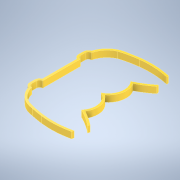
# Autodesk Inventor part: ovladac
Saved by Autodesk Inventor 2022 (Build 260153000, 153)
## iProperties
Created: 2022-12-02
Part Number: ovladac
Material: Generic
Document SubType Name: Modeling
Designer: matys
Density: 1 g/cm^3
Appearance: Glossy - Gold
Author: matys
Autodesk Inventor part; units mm, degrees
ref_plane "YZ Plane" through (0, 0, 0) normal (1, 0, 0) x (0, 1, 0)
ref_plane "XZ Plane" through (0, 0, 0) normal (0, 1, 0) x (-1, 0, 0)
ref_plane "XY Plane" through (0, 0, 0) normal (0, 0, 1) x (1, 0, 0)
sketch "Sketch1" plane through (0, 0, 0) normal (0, 1, 0) x (-1, 0, 0)
  circle A0 centre (0, 0) radius 17.5
  line L0 (0, -17.5) -> (0, -77.5)
  line L1 (0, -77.5) -> (0, -95)
  circle A1 centre (0, -95) radius 17.5
  line L2 (0, 0) -> (0, -25)
  line L3 (0, -25) -> (-22.5, -25)
  circle A2 centre (-22.5, -25) radius 12.5
  line L4 (-86.0476, -189.7218) -> (-86.0476, -216.7218)
  line L5 (-86.0476, -216.7218) -> (-52.0476, -216.7218)
  line L6 (-52.0476, -216.7218) -> (-52.0476, -189.7218)
  line L7 (-52.0476, -189.7218) -> (-86.0476, -189.7218)
  line L8 (-86.0476, -189.7218) -> (-52.0476, -216.7218)
  line L9 (-52.0476, -189.7218) -> (-86.0476, -216.7218)
  line L10 (0, -25) -> (0, -17.5)
  line L11 (0, -25) -> (0, -32.5)
  circle A3 centre (-22.5, -70) radius 12.5
  line L12 (-39.5, -56.5) -> (-39.5, -83.5)
  line L13 (-39.5, -83.5) -> (-5.5, -83.5)
  line L14 (-5.5, -83.5) -> (-5.5, -56.5)
  line L15 (-5.5, -56.5) -> (-39.5, -56.5)
  line L16 (-39.5, -56.5) -> (-5.5, -83.5)
  line L17 (-5.5, -56.5) -> (-39.5, -83.5)
  line L18 (-5.5, -56.5) -> (-22.5, -70)
  line L19 (-109.6323, -189.7218) -> (-115.6323, -189.7218)
  line L20 (-115.6323, -189.7218) -> (-115.6323, -195.7218)
  line L21 (-115.6323, -195.7218) -> (-109.6323, -195.7218)
  line L22 (-109.6323, -195.7218) -> (-109.6323, -189.7218)
  line L23 (-115.6323, -189.7218) -> (-109.6323, -195.7218)
  line L24 (-109.6323, -189.7218) -> (-115.6323, -195.7218)
  line L25 (0, -112.5) -> (0, -106)
  line L26 (-3, -109) -> (-3, -103)
  line L27 (-3, -103) -> (3, -103)
  line L28 (3, -103) -> (3, -109)
  line L29 (3, -109) -> (-3, -109)
  line L30 (14, -98) -> (8, -98)
  line L31 (14, -92) -> (14, -98)
  line L32 (8, -98) -> (8, -92)
  line L33 (8, -92) -> (14, -92)
  line L34 (3, -81) -> (3, -87)
  line L35 (-3, -81) -> (3, -81)
  line L36 (3, -87) -> (-3, -87)
  line L37 (-3, -87) -> (-3, -81)
  line L38 (-14, -92) -> (-8, -92)
  line L39 (-14, -98) -> (-14, -92)
  line L40 (-8, -92) -> (-8, -98)
  line L41 (-8, -98) -> (-14, -98)
  line L42 (-135.6088, -189.7218) -> (-135.6088, -214.7218)
  line L43 (-135.6088, -214.7218) -> (-162.6088, -214.7218)
  line L44 (-162.6088, -214.7218) -> (-162.6088, -189.7218)
  line L45 (-162.6088, -189.7218) -> (-135.6088, -189.7218)
  line L46 (-162.6088, -189.7218) -> (-135.6088, -214.7218)
  line L47 (-135.6088, -189.7218) -> (-162.6088, -214.7218)
  line L48 (17.5, 0) -> (17.5, -95)
  line L49 (-162.6088, -202.2218) -> (-135.6088, -202.2218)
  line L50 (25.5, -35) -> (25.5, -60)
  line L51 (25.5, -60) -> (-1.5, -60)
  line L52 (-1.5, -60) -> (-1.5, -35)
  line L53 (-1.5, -35) -> (25.5, -35)
  line L54 (25.5, -35) -> (20.5, -35)
  line L55 (20.5, -35) -> (20.5, -60)
  line L56 (-1.5, -35) -> (6.5, -35)
  line L57 (6.5, -35) -> (6.5, -60)
  line L58 (-1.5, -47.5) -> (6.5, -47.5)
  line L59 (-1.5, -35) -> (35.8, -35)
  line L60 (25.5, -60) -> (29.5, -60)
  line L61 (29.5, -60) -> (29.5, -47.5)
  line L62 (29.5, -47.5) -> (25.5, -47.5)
  line L63 (29.5, -60) -> (-7.8, -60)
  line L64 (-7.8, -60) -> (-7.8, -35)
  line L65 (-7.8, -35) -> (-1.5, -35)
  dimension "d0" = 35
  dimension "d1" = 60
  dimension "d2" = 17.5
  dimension "d3" = 25
  dimension "d4" = 22.5
  dimension "d6" = 25
  dimension "d7" = 27
  dimension "d8" = 34
  dimension "d9" = 27
  dimension "d10" = 7.5
  dimension "d11" = 25
  dimension "d12" = 27
  dimension "d13" = 34
  dimension "d14" = 27
  dimension "d15" = 6
  dimension "d16" = 6
  dimension "d17" = 6
  dimension "d18" = 6.5
  dimension "d22" = 6
  dimension "d25" = 360
  dimension "d27" = 25
  dimension "d28" = 27
  dimension "d32" = 25
  dimension "d33" = 27
  dimension "d34" = 5
  dimension "d35" = 8
  dimension "d36" = 8
  dimension "d72" = 37.3
  dimension "d73" = 4
  dimension "d74" = 37.3
  constraints: 132 end point, 20 perpendicular, 8 point on line, 8 vertical, 6 midpoint, 5 point on circle, 4 centre point, 3 coincident, 3 horizontal, 1 collinear, 1 tangent, 33 other
  measures "d0" diameter of A0
  measures "d1" distance of L0.start L0.end
  measures "d2" distance of L0.end L1.end
  measures "d3" distance of L2.start L2.end
  measures "d4" distance of L2.end L3.end
  measures "d6" diameter of A2
  measures "d7" distance of L4.start L4.end
  measures "d8" distance of L4.end L5.end
  measures "d9" distance of L5.end L6.end
  measures "d10" distance of L2.end L11.end
  measures "d11" diameter of A3
  measures "d12" distance of L15.end L12.end
  measures "d13" distance of L12.end L14.start
  measures "d14" distance of L14.start L15.start
  measures "d15" distance of L19.start L19.end
  measures "d16" distance of L19.end L20.end
  measures "d17" distance of L20.end L21.end
  measures "d18" distance of L25.start L25.end
  measures "d22" distance of L26.start L26.end
  measures "d27" distance of L42.start L42.end
  measures "d28" distance of L42.end L43.end
  measures "d32" distance of L50.start L50.end
  measures "d33" distance of L50.end L51.end
  measures "d34" distance of L50.start L54.end
  measures "d35" distance of L52.end L56.end
  measures "d36" distance between parallel lines of L50 L48
  measures "d72" distance of L52.end L59.end
  measures "d73" distance of L50.end L60.end
  measures "d74" distance of L60.end L63.end
sketch "Sketch2" plane through (0, 0, 0) normal (0, 1, 0) x (-1, 0, 0)
  circle A0 centre (0, 0) radius 17.5
  line L0 (0, 17.5) -> (0, 25.5)
  line L1 (17.5, 0) -> (29.5, 0)
  line L2 (0, 0) -> (0, 17.5)
  line L3 (0, 17.5) -> (17.5, 0)
  line L4 (0, 0) -> (8.75, 8.75)
  line L5 (8.75, 8.75) -> (12.3744, 12.3744)
  line L6 (12.3744, 12.3744) -> (18.0312, 18.0312)
  arc A1 (29.5, 0) -> (10.5727, 22.6518) centre (-3.4308, -8.2827) ccw
  line L7 (0, -20.5) -> (0, -80.5)
  line L8 (0, -80.5) -> (0, -98)
  line L9 (29.5, 0) -> (29.5, -17.5) construction
  line L10 (34.5, -12.5) -> (34.5, -5)
  arc A2 (34.5, -5) -> (29.5, 0) centre (29.5, -5) ccw
  arc A3 (29.5, -17.5) -> (34.5, -12.5) centre (29.5, -12.5) ccw
  line L11 (29.5, -17.5) -> (29.5, -47.5)
  line L12 (0, -20.5) -> (0, -25.5)
  line L13 (0, -17.5) -> (0, -21.5)
  line L14 (0, -17.5) -> (0, -25)
  line L15 (0, -25) -> (-22.5, -25)
  circle A4 centre (-22.5, -25) radius 12.5
  line L16 (-9, -8) -> (-36, -8)
  line L17 (-36, -8) -> (-36, -42)
  line L18 (-36, -42) -> (-9, -42)
  line L19 (-9, -42) -> (-9, -8)
  line L20 (-36, -42) -> (-9, -8)
  line L21 (-36, -8) -> (-9, -42)
  line L22 (-22.5, -25) -> (-36, -42)
  line L23 (0, -17.5) -> (0, -11)
  line L24 (0, -11) -> (3, -11)
  line L25 (3, -11) -> (3, -8)
  line L26 (3, -8) -> (-3, -8)
  line L27 (-3, -8) -> (-3, -14)
  line L28 (-3, -14) -> (3, -14)
  line L29 (3, -14) -> (3, -11)
  line L30 (14, 3) -> (11, 3)
  line L31 (8, 3) -> (8, -3)
  line L32 (11, 3) -> (8, 3)
  line L33 (8, -3) -> (14, -3)
  line L34 (14, -3) -> (14, 3)
  line L35 (-3, 14) -> (-3, 11)
  line L36 (-3, 8) -> (3, 8)
  line L37 (-3, 11) -> (-3, 8)
  line L38 (3, 8) -> (3, 14)
  line L39 (3, 14) -> (-3, 14)
  line L40 (-14, -3) -> (-11, -3)
  line L41 (-8, -3) -> (-8, 3)
  line L42 (-11, -3) -> (-8, -3)
  line L43 (-8, 3) -> (-14, 3)
  line L44 (-14, 3) -> (-14, -3)
  line L45 (0, -47.5) -> (-33.3972, -47.5)
  arc A5 (-41.1706, -8.3745) -> (-33.3972, -47.5) centre (-22.5, -25) ccw
  arc A6 (10.5727, -117.6518) -> (29.5, -95) centre (-3.4308, -86.7173) ccw
  line L46 (34.5, -82.5) -> (34.5, -90)
  arc A7 (29.5, -95) -> (34.5, -90) centre (29.5, -90) ccw
  arc A8 (34.5, -82.5) -> (29.5, -77.5) centre (29.5, -82.5) ccw
  line L47 (29.5, -77.5) -> (29.5, -47.5)
  ellipse E0 centre (-5.5218, -98.3783) end of major axis (-65.9225, -112.4065) minor radius 22.7978 (-28.0257, -81.2123) -> (10.5727, -117.6518) ccw
  arc A9 (-33.3972, -47.5) -> (-41.1706, -86.6255) centre (-22.5, -70) ccw
  line L48 (0, -95) -> (0, -112.5)
  line L49 (-9, -87) -> (-36, -87)
  line L50 (-36, -87) -> (-36, -53)
  line L51 (-36, -53) -> (-9, -53)
  line L52 (-9, -53) -> (-9, -87)
  line L53 (0, -77.5) -> (0, -84)
  line L54 (0, -84) -> (3, -84)
  line L55 (3, -84) -> (3, -87)
  line L56 (3, -87) -> (-3, -87)
  line L57 (-3, -87) -> (-3, -81)
  line L58 (-3, -81) -> (3, -81)
  line L59 (3, -81) -> (3, -84)
  line L60 (14, -98) -> (11, -98)
  line L61 (8, -98) -> (8, -92)
  line L62 (11, -98) -> (8, -98)
  line L63 (8, -92) -> (14, -92)
  line L64 (14, -92) -> (14, -98)
  line L65 (-3, -109) -> (-3, -106)
  line L66 (-3, -103) -> (3, -103)
  line L67 (-3, -106) -> (-3, -103)
  line L68 (3, -103) -> (3, -109)
  line L69 (3, -109) -> (-3, -109)
  line L70 (-14, -92) -> (-11, -92)
  line L71 (-8, -92) -> (-8, -98)
  line L72 (-11, -92) -> (-8, -92)
  line L73 (-8, -98) -> (-14, -98)
  line L74 (-14, -98) -> (-14, -92)
  line L75 (0, -47.5) -> (-1.5, -47.5)
  line L76 (-1.5, -47.5) -> (-1.5, -60)
  line L77 (-1.5, -60) -> (25.5, -60)
  line L78 (25.5, -60) -> (25.5, -35)
  line L79 (25.5, -35) -> (-1.5, -35)
  line L80 (-1.5, -35) -> (-1.5, -47.5)
  line L81 (0, -17.5) -> (0, -25)
  line L82 (0, -47.5) -> (0, -35)
  line L83 (25.5, -44.7664) -> (24.099, -44.7664)
  line L84 (-5.5218, 3.3783) -> (-65.9225, 17.4065)
  line L85 (-5.5218, 3.3783) -> (-5.5218, 9.5)
  line L86 (-65.9225, 17.4065) -> (128.8922, -27.8397)
  line L87 (0, 0) -> (0, -15)
  line L88 (0, -15) -> (15, -15)
  line L89 (15, -15) -> (15, 15)
  line L90 (15, 15) -> (-15, 15)
  line L91 (-15, 15) -> (-15, -15)
  line L92 (0, -15) -> (-15, -15)
  line L93 (-65.9225, 17.4065) -> (-19.167, 6.5474)
  line L94 (-19.167, 6.5474) -> (-21.2031, -2.2192)
  line L95 (-21.2031, -2.2192) -> (-67.9586, 8.6399)
  line L96 (-67.9586, 8.6399) -> (-65.9225, 17.4065)
  line L97 (-65.9225, 17.4065) -> (-63.8865, 26.1732)
  line L98 (-63.8865, 26.1732) -> (-17.1309, 15.3141)
  line L99 (-17.1309, 15.3141) -> (-19.167, 6.5474)
  line L100 (-21.2031, -2.2192) -> (-28.0257, -13.7877)
  line L101 (-28.0257, -13.7877) -> (-21.0551, 16.2255)
  arc A10 (-67.9586, 8.6399) -> (-28.0257, -13.7877) centre (15.2695, 110.0655) ccw
  line L102 (-28.0257, -13.7877) -> (-21.0551, 16.2255)
  arc A11 (-18.1566, 28.7053) -> (-63.8865, 26.1732) centre (-33.8791, -101.5517) ccw
  line L103 (-63.8865, 26.1732) -> (-65.0129, 25.9033)
  line L104 (-67.9586, 8.6399) -> (-68.8508, 9.3786)
  ellipse E1 centre (-65.9225, 17.4065) end of major axis (-63.8865, 26.1732) minor radius 3.0998 (-67.9586, 8.6399) -> (-63.8865, 26.1732) ccw
  ellipse E2 centre (-65.9225, 17.4065) end of major axis (-63.8865, 26.1732) minor radius 3.0998 (-65.0129, 25.9033) -> (-68.8508, 9.3786) ccw
  line L105 (-67.9586, 8.6399) -> (-67.2799, 11.5621)
  line L106 (-67.2799, 11.5621) -> (-64.3577, 10.8834)
  line L107 (-64.3577, 10.8834) -> (-65.0364, 7.9612)
  line L108 (-63.8865, 26.1732) -> (-64.5652, 23.251)
  line L109 (-64.5652, 23.251) -> (-63.8865, 26.1732)
  line L110 (-63.8865, 26.1732) -> (-60.9642, 25.4945)
  line L111 (-60.9642, 25.4945) -> (-61.6429, 22.5723)
  line L112 (-61.6429, 22.5723) -> (-64.5652, 23.251)
  line L113 (0, -80) -> (15, -80)
  line L114 (15, -80) -> (15, -110)
  line L115 (15, -110) -> (-15, -110)
  line L116 (-15, -110) -> (-15, -80)
  line L117 (0, -80) -> (-15, -80)
  arc A12 (-28.0257, -81.2123) -> (-67.9586, -103.6399) centre (15.2695, -205.0655) ccw
  arc A13 (-63.8865, -121.1732) -> (-18.1566, -123.7053) centre (-33.8791, 6.5517) ccw
  line L118 (-63.8865, -121.1732) -> (-65.0129, -120.9033)
  line L119 (-67.9586, -103.6399) -> (-68.8508, -104.3786)
  ellipse E3 centre (-65.9225, -112.4065) end of major axis (-63.8865, -121.1732) minor radius 3.0998 (-68.8508, -104.3786) -> (-65.0129, -120.9033) ccw
  line L120 (0, -47.5) -> (6.5, -47.5)
  line L121 (6.5, -47.5) -> (6.5, -60)
  line L122 (6.5, -60) -> (6.5, -80)
  line L123 (6.5, -70) -> (6.5, -60)
  line L124 (6.5, -60) -> (20.5, -60)
  line L125 (20.5, -60) -> (20.5, -70)
  line L126 (20.5, -70) -> (6.5, -70)
  line L127 (6.5, -70) -> (6.5, -67)
  line L128 (6.5, -67) -> (8, -67)
  line L129 (8, -67) -> (8, -70)
  line L130 (8, -67) -> (20.5, -67)
  line L131 (20.5, -67) -> (19, -67)
  line L132 (19, -67) -> (19, -70)
  line L133 (6.5, -60) -> (6.5, -70)
  line L134 (6.5, -70) -> (6.5, -73)
  line L135 (6.5, -73) -> (19, -73)
  line L136 (19, -73) -> (19, -70)
  line L137 (8, -73) -> (8, -70)
  line L138 (19, -70) -> (8, -70)
  line L139 (8, -28) -> (8, -25)
  line L140 (8, -28) -> (20.5, -28)
  line L141 (19, -28) -> (19, -25)
  line L142 (6.5, -22) -> (19, -22)
  line L143 (19, -22) -> (19, -25)
  line L144 (8, -22) -> (8, -25)
  line L145 (25.5, -60) -> (25.5, -73)
  line L146 (25.5, -73) -> (19, -73)
  ellipse E4 centre (-5.5218, 3.3783) end of major axis (-65.9225, 17.4065) minor radius 22.7978 (10.5727, 22.6518) -> (-18.1566, 28.7053) ccw
  ellipse E5 centre (-5.5218, 3.3783) end of major axis (-65.9225, 17.4065) minor radius 22.7978 (-58.9806, 25.0338) -> (-64.5851, 9.9042) ccw
  ellipse E6 centre (-5.5218, 3.3783) end of major axis (-65.9225, 17.4065) minor radius 22.7978 (-63.0527, 7.5005) -> (-28.0257, -13.7877) ccw
  arc A14 (-17.8019, 31.6843) -> (-63.1315, 29.4239) centre (-33.8791, -101.5517) ccw
  line L147 (-18.1328, 15.5468) -> (-25.1035, -14.4663)
  arc A15 (31.8748, 2.6394) -> (0.4994, 28.4642) centre (-3.4308, -8.2827) ccw
  line L148 (25.5, -47.5) -> (29.5, -47.5)
  line L149 (32.5, -47.5) -> (32.5, -19.9162)
  arc A16 (32.5, -19.9162) -> (37.5, -12.5) centre (29.5, -12.5) ccw
  line L150 (37.5, -12.5) -> (37.5, -5)
  arc A17 (37.5, -5) -> (31.8748, 2.6394) centre (29.5, -5) ccw
  line L151 (-65.9225, 17.4065) -> (-63.1315, 29.4239)
  arc A18 (-68.7136, 5.3892) -> (-45.7824, -9.4458) centre (15.2695, 110.0655) ccw
  arc A19 (-43.9451, -6.997) -> (-43.9554, -7.0092) centre (-22.5, -25) ccw
  arc A20 (-45.7824, -9.4458) -> (-39.1658, -47.5) centre (-22.5, -25) ccw
  line L152 (-65.9225, 17.4065) -> (-68.7136, 5.3892)
  arc A21 (-45.7824, -85.5542) -> (-68.7136, -100.3892) centre (15.2695, -205.0655) ccw
  arc A22 (-39.1658, -47.5) -> (-45.7824, -85.5542) centre (-22.5, -70) ccw
  line L153 (-65.9225, -112.4065) -> (-68.7136, -100.3892)
  arc A23 (-63.1315, -124.4239) -> (-17.8019, -126.6843) centre (-33.8791, 6.5517) ccw
  arc A24 (0.4994, -123.4642) -> (31.8748, -97.6394) centre (-3.4308, -86.7173) ccw
  line L154 (32.5, -47.5) -> (32.5, -75.0838)
  arc A25 (37.5, -82.5) -> (32.5, -75.0838) centre (29.5, -82.5) ccw
  line L155 (37.5, -82.5) -> (37.5, -90)
  arc A26 (31.8748, -97.6394) -> (37.5, -90) centre (29.5, -90) ccw
  line L156 (-65.9225, -112.4065) -> (-63.1315, -124.4239)
  arc A27 (-17.8019, -126.6843) -> (0.4994, -123.4642) centre (-51.4005, 117.889) ccw
  spline S0 degree 5 poles (-17.8067, 31.6848) (-14.1127, 31.2511) (-10.4318, 30.7055) (-6.7676, 30.0569) (-3.1227, 29.3096) (0.4994, 28.4642) knots 0 0 0 0 0 0 1 1 1 1 1 1
  point P0 (29.5, -8.75)
  point P1 (0, -35)
  point P2 (0, -60)
  point P3 (-9.0139, -15)
  point P4 (-9, -15.0083)
  point P5 (-15.5644, -8)
  point P6 (-15, -9.0139)
  point P7 (-41.1721, -8.3761)
  point P8 (-62.9032, 16.7053)
  point P9 (-25.1272, -1.3078)
  point P10 (-21.0551, 16.2255)
  point P11 (-15, -87)
  point P12 (-36, -84.2978)
  point P13 (-9, -80)
  point P14 (-30.0534, -124.595)
  point P15 (-41.1721, -86.6239)
  point P16 (-25.1272, -1.3078)
  point P17 (-21.0551, 16.2255)
  point P18 (-15, -8)
  point P19 (-36.4689, -49.2667)
  point P20 (-36.4689, -45.7333)
  point P21 (-23.0911, 7.4588)
  point P22 (-23.0911, 7.4588)
  point P23 (-30.0534, -124.595)
  point P24 (-39.0969, -85.6571)
  point P25 (-18.1566, -123.7053)
  point P26 (-18.1566, 28.7053)
  point P27 (-67.9586, -103.6399)
  dimension "d93" = 3
  dimension "d37" = 35
  dimension "d38" = 8
  dimension "d39" = 12
  dimension "d40" = 8
  dimension "d41" = 60
  dimension "d42" = 17.5
  dimension "d47" = 4
  dimension "d48" = 7.5
  dimension "d49" = 22.5
  dimension "d50" = 25
  dimension "d51" = 27
  dimension "d52" = 34
  dimension "d53" = 6.5
  dimension "d54" = 3
  dimension "d55" = 3
  dimension "d56" = 6
  dimension "d57" = 6
  dimension "d60" = 360
  dimension "d65" = 1.5
  dimension "d66" = 12.5
  dimension "d67" = 27
  dimension "d68" = 25
  dimension "d69" = 1.401
  dimension "d70" = 76.925
  dimension "d71" = 200
  dimension "d75" = 15
  dimension "d76" = 15
  dimension "d77" = 30
  dimension "d78" = 30
  dimension "d79" = 48
  dimension "d80" = 9
  dimension "d81" = 9
  dimension "d82" = 3
  dimension "d83" = 3
  dimension "d84" = 3
  dimension "d85" = 3
  dimension "d86" = 6.5
  dimension "d87" = 14
  dimension "d88" = 3
  dimension "d89" = 1.5
  dimension "d90" = 1.5
  dimension "d91" = 3
  dimension "d92" = 3
  dimension "d94" = 3
  constraints: 316 end point, 80 symmetric about line, 66 point on circle, 59 point on line, 38 perpendicular, 28 centre point, 6 vertical, 5 horizontal, 5 midpoint, 4 coincident, 4 collinear, 3 parallel, 2 tangent, 101 other
  measures "d37" diameter of A0
  measures "d38" distance of L0.start L0.end
  measures "d39" distance of L1.end L1.start
  measures "d40" distance of L5.end L6.end
  measures "d41" distance of L7.start L7.end
  measures "d42" distance of L7.end L8.end
  measures "d47" distance of L13.start L13.end
  measures "d48" distance of L13.start L14.end
  measures "d49" distance of L14.end L15.end
  measures "d50" diameter of A4
  measures "d51" distance of L16.start L16.end
  measures "d52" distance of L16.end L17.end
  measures "d53" distance of L13.start L23.end
  measures "d54" distance of L23.end L24.end
  measures "d55" distance of L24.end L25.end
  measures "d56" distance of L25.end L26.end
  measures "d57" distance of L26.end L27.end
  measures "d65" distance of L45.start L75.end
  measures "d66" distance of L75.end L76.end
  measures "d67" distance of L76.end L77.end
  measures "d68" distance of L77.end L78.end
  measures "d69" distance of L83.start L83.end
  measures "d70" angle of L85 L84
  measures "d71" distance of L86.start L86.end
  measures "d75" distance of L2.start L87.end
  measures "d76" distance of L87.end L88.end
  measures "d77" distance of L88.end L89.end
  measures "d78" distance of L89.end L90.end
  measures "d79" distance of L86.start L93.end
  measures "d80" distance of L93.end L94.end
  measures "d81" distance of L84.end L97.end
  measures "d82" distance of L95.end L105.end
  measures "d83" distance of L105.end L106.end
  measures "d84" distance of L97.end L108.end
  measures "d85" distance of L97.end L110.end
  measures "d86" distance of L45.start L120.end
  measures "d87" distance of L121.end L124.end
  measures "d88" distance of L123.start L127.end
  measures "d89" distance of L127.end L128.end
  measures "d90" distance of L130.end L131.end
  measures "d91" distance of L123.start L134.end
  measures "d92" radial gap between concentric circles of A11 A14
  measures "d94" distance between parallel lines of L11 L149
extrude "Extrusion1" add sketch "Sketch2" along normal blind 10 contours A1 E4 A11 L151 A14 S0 A15 A17 L150 L86 L10 A2 | L86 L150 A16 L149 L154 A25 L155 A26 A24 A27 A23 L156 A13 E0 A6 A7 L46 A8 L47 L11 A3 L10 | A10 A5 A9 A12 L153 A21 A22 A20 A18 L152
body "Solid1"
